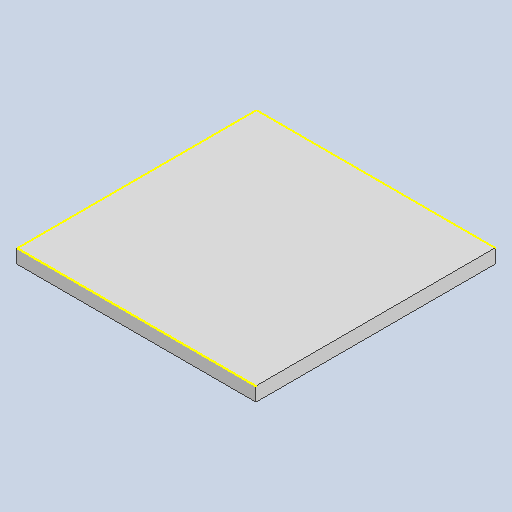
# Autodesk Inventor part: rubber
Saved by Autodesk Inventor 2024.3 (Build 283343000, 343)
## iProperties
Created: 2024-11-17
Part Number: rubber
Material: Generic
Document SubType Name: Modeling
Designer: Ryba
Density: 1 g/cm^3
Appearance: Default
Author: Ryba
Autodesk Inventor part; units mm, degrees
ref_plane "YZ Plane" through (0, 0, 0) normal (1, 0, 0) x (0, 1, 0)
ref_plane "XZ Plane" through (0, 0, 0) normal (0, 1, 0) x (-1, 0, 0)
ref_plane "XY Plane" through (0, 0, 0) normal (0, 0, 1) x (1, 0, 0)
sketch "Sketch1" plane through (0, 0, 0) normal (0, 1, 0) x (-1, 0, 0)
  line L0 (0, 0) -> (0, -17)
  line L1 (0, -17) -> (17, -17)
  line L2 (17, -17) -> (17, 0)
  line L3 (17, 0) -> (0, 0)
  dimension "d0" = 17
  dimension "d1" = 17
  constraints: 8 end point, 3 perpendicular, 1 vertical
  measures "d0" distance of L0.start L0.end
  measures "d1" distance of L0.end L1.end
extrude "Extrusion1" add sketch "Sketch1" along normal blind 1
sketch "Sketch2" plane through (0, 1, 0) normal (0, 1, 0) x (1, 0, 0)
  line L0 (-17, 17) -> (-17, 0) projected
  line L1 (0, 17) -> (-17, 17) projected
  line L2 (-17, 0) -> (0, 0) projected
body "Solid1"
